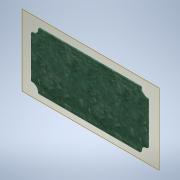
# Autodesk Inventor part: PCB
Saved by Autodesk Inventor 2021 (Build 250183000, 183)
## iProperties
Created: 2021-04-07
Part Number: PCB
Material: Generic
Document SubType Name: Modeling
Designer: James
Density: 1 g/cm^3
Appearance: Green Polished
Author: James
Autodesk Inventor part; units mm, degrees
ref_plane "YZ Plane" through (0, 0, 0) normal (1, 0, 0) x (0, 1, 0)
ref_plane "XZ Plane" through (0, 0, 0) normal (0, 1, 0) x (-1, 0, 0)
ref_plane "XY Plane" through (0, 0, 0) normal (0, 0, 1) x (1, 0, 0)
ref_plane "Work Plane1" through (0, 0, 0) normal (0, 0, 1) x (1, 0, 0)
sketch "Sketch1" plane through (0, 0, 0) normal (0, 0, 1) x (1, 0, 0)
  arc A0 (-65.0831, -34.4583) -> (-71.9583, -27.5831) centre (-71.818, -34.318) ccw
  line L0 (-74, -25.5835) -> (-74, 25.5835)
  arc A1 (-71.9583, 27.5831) -> (-65.0831, 34.4583) centre (-71.818, 34.318) ccw
  line L1 (-63.0835, 36.5) -> (63.0835, 36.5)
  arc A2 (65.0831, 34.4583) -> (71.9583, 27.5831) centre (71.818, 34.318) ccw
  line L2 (74, 25.5835) -> (74, -25.5835)
  arc A3 (71.9583, -27.5831) -> (65.0831, -34.4583) centre (71.818, -34.318) ccw
  line L3 (63.0835, -36.5) -> (-63.0835, -36.5)
  arc A4 (-65.0831, -34.4583) -> (-71.9583, -27.5831) centre (-71.818, -34.318) ccw
  circle A5 centre (-58.0835, -31.5) radius 1.25 projected
  circle A6 centre (-69, 0) radius 1.25 projected
  circle A7 centre (-58.0835, 31.5) radius 1.25 projected
  circle A8 centre (-58.0835, 31.5) radius 1.25 projected
  circle A9 centre (0, 31.5) radius 1.25 projected
  circle A10 centre (58.0835, 31.5) radius 1.25
  circle A11 centre (69, 0) radius 1.25 projected
  circle A12 centre (58.0835, -31.5) radius 1.25 projected
  circle A13 centre (0, -31.5) radius 1.25
  line L4 (-73, -25.5835) -> (-73, 25.5835) construction
  arc A14 (-71.9792, 26.5833) -> (-64.0833, 34.4792) centre (-71.818, 34.318) ccw
  line L5 (-63.0835, 35.5) -> (63.0835, 35.5) construction
  arc A15 (-71.9792, 26.5833) -> (-73, 25.5835) centre (-72, 25.5835) ccw
  arc A16 (-63.0835, 35.5) -> (-64.0833, 34.4792) centre (-63.0835, 34.5) ccw
  line L6 (-73, 25.5835) -> (-73, 0)
  line L7 (-63.0835, 35.5) -> (0, 35.5)
  line L8 (-78, 0) -> (78, 0) projected
  line L9 (0, 40.5) -> (0, -40.5) projected
  arc A17 (-64.0833, -34.4792) -> (-71.9792, -26.5833) centre (-71.818, -34.318) ccw
  arc A18 (-73, -25.5835) -> (-71.9792, -26.5833) centre (-72, -25.5835) ccw
  arc A19 (-64.0833, -34.4792) -> (-63.0835, -35.5) centre (-63.0835, -34.5) ccw
  line L10 (-73, -25.5835) -> (-73, 0)
  line L11 (-63.0835, -35.5) -> (0, -35.5)
  arc A20 (64.0833, 34.4792) -> (71.9792, 26.5833) centre (71.818, 34.318) ccw
  arc A21 (73, 25.5835) -> (71.9792, 26.5833) centre (72, 25.5835) ccw
  arc A22 (64.0833, 34.4792) -> (63.0835, 35.5) centre (63.0835, 34.5) ccw
  line L12 (73, 25.5835) -> (73, 0)
  line L13 (63.0835, 35.5) -> (0, 35.5)
  line L14 (73, -25.5835) -> (73, 0)
  arc A23 (71.9792, -26.5833) -> (73, -25.5835) centre (72, -25.5835) ccw
  arc A24 (71.9792, -26.5833) -> (64.0833, -34.4792) centre (71.818, -34.318) ccw
  arc A25 (63.0835, -35.5) -> (64.0833, -34.4792) centre (63.0835, -34.5) ccw
  line L15 (63.0835, -35.5) -> (0, -35.5)
  point P0 (0, 0)
  dimension "board_clearance" = 1
  dimension "d1" = 1
  dimension "d2" = 1
  constraints: 34 point on circle, 28 end point, 21 symmetric about line, 19 centre point, 2 coincident, 2 horizontal, 2 midpoint, 2 parallel, 2 tangent, 2 vertical, 39 other
  measures "board_clearance" distance between parallel lines of L0 L4
  measures "d1" radial gap between concentric circles of A1 A14
  measures "d2" distance between parallel lines of L1 L5
extrude "Extrusion1" add sketch "Sketch1" along normal blind 1.6 contours L8 L9 A13 L11 A19 A17 A18 L10 A6 | A6 L8 L6 A15 A14 A16 L7 L9 A9 | L9 A9 L13 A22 A20 A21 L12 L8 A11 | L8 A11 L14 A23 A24 A25 L15 L9 A13
equation "\"d1\" = board_clearance"
equation "\"d2\" = board_clearance"
body "Solid1"
